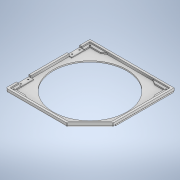
# Autodesk Inventor part: Box_Walls_2
Saved by Autodesk Inventor 2022 (Build 260153000, 153)
## iProperties
Created: 2023-02-27
Part Number: Box_Walls_2
Material: Generic
Document SubType Name: Modeling
Designer: zarek
Density: 1 g/cm^3
Appearance: Default
Author: zarek
Autodesk Inventor part; units mm, degrees
ref_plane "YZ Plane" through (0, 0, 0) normal (1, 0, 0) x (0, 1, 0)
ref_plane "XZ Plane" through (0, 0, 0) normal (0, 1, 0) x (-1, 0, 0)
ref_plane "XY Plane" through (0, 0, 0) normal (0, 0, 1) x (1, 0, 0)
sketch "Sketch1" plane through (0, 0, 0) normal (0, 1, 0) x (-1, 0, 0)
  line L0 (101.6, -101.6) -> (-101.6, -101.6)
  line L1 (-101.6, -101.6) -> (-101.6, 101.6)
  line L2 (-101.6, 101.6) -> (101.6, 101.6)
  line L3 (101.6, 101.6) -> (101.6, -101.6)
  line L4 (96.6, -96.6) -> (-96.6, -96.6)
  line L5 (-96.6, -96.6) -> (-96.6, 96.6)
  line L6 (-96.6, 96.6) -> (96.6, 96.6)
  line L7 (96.6, 96.6) -> (96.6, -96.6)
  line L8 (101.6, 101.6) -> (-40.4, 101.6)
  circle A0 centre (0, 0) radius 88.9
  circle A1 centre (0, 0) radius 109.3376
  line L9 (-40.4, 101.6) -> (-101.6, 40.4)
  line L10 (-45.4, 101.6) -> (-101.6, 45.4)
  line L11 (96.6, 96.6) -> (96.6, 101.6)
  line L12 (-45.4, 101.6) -> (-35.4, 101.6)
  line L13 (-35.4, 101.6) -> (-35.4, 96.6)
  line L14 (-35.4, 96.6) -> (-45.4, 96.6)
  line L15 (-45.4, 96.6) -> (-45.4, 101.6)
  circle A2 centre (0, 0) radius 111.3376
  point P0 (96.6, 51.2168)
  point P1 (101.6, 40.4)
  point P2 (101.6, -40.4)
  point P3 (96.6, -51.2168)
  point P4 (-96.6, 45.4)
  point P5 (-45.4, 96.6)
  dimension "d0" = 203.2
  dimension "d1" = 203.2
  dimension "d2" = 101.6
  dimension "d3" = 101.6
  dimension "d4" = 5
  dimension "d5" = 5
  dimension "d6" = 5
  dimension "d7" = 5
  dimension "d10" = 142
  dimension "d12" = 61.2
  dimension "d14" = 177.8
  dimension "d15" = 5
  dimension "d16" = 5
  dimension "d17" = 10
  dimension "d34" = 2
  constraints: 32 end point, 7 parallel, 6 point on line, 4 perpendicular, 3 centre point, 3 coincident, 3 horizontal, 2 point on circle
  measures "d0" distance between parallel lines of L2 L0
  measures "d1" distance between parallel lines of L1 L3
  measures "d2" distance from line of L0 point (0, 0)
  measures "d3" distance from line of L1 point (0, 0)
  measures "d4" distance between parallel lines of L4 L0
  measures "d5" distance between parallel lines of L1 L5
  measures "d6" distance between parallel lines of L2 L6
  measures "d7" distance between parallel lines of L3 L7
  measures "d10" distance of L2.end L8.end
  measures "d12" distance from line of L1 L8.end
  measures "d14" diameter of A0
  measures "d15" distance of L10.end L9.end
  measures "d16" distance of L10.start L8.end
  measures "d17" distance of L13.end L14.end
  measures "d34" radial gap between concentric circles of A1 A2
extrude "Extrusion1" add sketch "Sketch1" along normal blind 3 contours L0 A2 L4 L7 L3 | L0 A1 L4 A2 | A2 L7 A1 L3 | L0 A1 L4 | A2 L4 A1 L0 | L0 L1 A2 L5 L4 | A2 L7 L4 | L4 A1 L7 A2 | A1 L7 L3 | L4 A1 L5 L9 L6 L7 | A2 L5 A1 L4 | L4 L5 A2 | A1 L7 A2 L3 | A2 L7 L11 L2 L3 | L1 A1 L5 A2 | A1 L6 A2 L7 | A2 L6 L7 | A1 L1 L9 L5 | A1 L2 A2 L6 | L6 L13 L2 A1 | L11 L6 A2 L2 | L9 A1 L10 L5 | L5 L10 L6 L9 | L1 L10 A1 | L6 L9 L2 L13 | L15 A1 L9 | L6 L10 A1 L15 | A1 L15 L2 | A1 L10 L15
sketch "Sketch5" plane through (0, 3, 0) normal (0, 1, 0) x (1, 0, 0)
  line L0 (-101.6, 101.6) -> (101.6, 101.6)
  line L1 (101.6, 101.6) -> (101.6, -101.6)
  line L2 (101.6, -101.6) -> (-101.6, -101.6)
  line L3 (-101.6, -101.6) -> (-101.6, 101.6)
  line L4 (-96.6, 96.6) -> (96.6, 96.6)
  line L5 (96.6, 96.6) -> (96.6, -96.6)
  line L6 (96.6, -96.6) -> (-96.6, -96.6)
  line L7 (-96.6, -96.6) -> (-96.6, 96.6)
  line L8 (-101.6, -101.6) -> (40.4, -101.6)
  circle A0 centre (0, 0) radius 88.9
  circle A1 centre (0, 0) radius 109.3376
  line L9 (40.4, -101.6) -> (101.6, -40.4)
  line L10 (45.4, -101.6) -> (101.6, -45.4)
  line L11 (-96.6, -96.6) -> (-96.6, -101.6)
  line L12 (45.4, -101.6) -> (35.4, -101.6)
  line L13 (35.4, -101.6) -> (35.4, -96.6)
  line L14 (35.4, -96.6) -> (45.4, -96.6)
  line L15 (45.4, -96.6) -> (45.4, -101.6)
  circle A2 centre (0, 0) radius 111.3376
  point P0 (96.6, 101.6)
  point P1 (96.6, 51.2168)
  point P2 (101.6, 40.4)
  point P3 (101.6, -40.4)
  point P4 (96.6, -51.2168)
  point P5 (-96.6, 45.4)
  point P6 (-45.4, 96.6)
  point P7 (-35.4, 101.6)
  point P8 (-55.358, -96.6)
  point P9 (-96.6, -55.358)
  point P10 (-96.6, 55.358)
  point P11 (-55.358, 96.6)
  point P12 (55.358, 96.6)
  point P13 (96.6, 55.358)
  point P14 (96.6, -45.4)
  point P15 (45.4, -96.6)
  dimension "d37" = 203.2
  dimension "d38" = 203.2
  dimension "d39" = 101.6
  dimension "d40" = 101.6
  dimension "d41" = 5
  dimension "d42" = 5
  dimension "d43" = 5
  dimension "d44" = 5
  dimension "d45" = 142
  dimension "d46" = 61.2
  dimension "d47" = 177.8
  dimension "d48" = 5
  dimension "d49" = 5
  dimension "d50" = 10
  dimension "d51" = 2
  constraints: 32 end point, 7 parallel, 6 point on line, 4 perpendicular, 3 centre point, 3 coincident, 2 point on circle
  measures "d37" distance between parallel lines of L2 L0
  measures "d38" distance between parallel lines of L1 L3
  measures "d39" distance from line of L0 point (0, 0)
  measures "d40" distance from line of L1 point (0, 0)
  measures "d41" distance between parallel lines of L4 L0
  measures "d42" distance between parallel lines of L1 L5
  measures "d43" distance between parallel lines of L2 L6
  measures "d44" distance between parallel lines of L3 L7
  measures "d45" distance of L2.end L8.end
  measures "d46" distance from line of L1 L8.end
  measures "d47" diameter of A0
  measures "d48" distance of L10.end L9.end
  measures "d49" distance of L10.start L8.end
  measures "d50" distance of L13.end L14.end
  measures "d51" radial gap between concentric circles of A1 A2
extrude "Extrusion4" add sketch "Sketch5" along normal blind 3 contours L0 A2 L4 L7 L3 | L0 A1 L4 A2 | A2 L7 A1 L3 | L0 A1 L4 | A2 L4 A1 L0 | L0 L1 A2 L5 L4 | A2 L7 L4 | A1 L7 L3 | A2 L7 L11 L2 L3 | L3 A1 L7 A2 | L4 L5 A2 | A2 L6 L7 | L1 A1 L5 A2 | L11 L6 A2 L2 | L6 A1 L2 A2 | A1 L1 L9 L5 | L6 L13 L2 A1 | L9 A1 L10 L5 | L5 L10 L6 L9 | L1 L10 A1 | L6 L9 L2 L13 | L15 A1 L9 | L6 L10 A1 L15 | A1 L15 L2 | L15 A1 L10
sketch "Sketch6" plane through (0, 6, 0) normal (0, 1, 0) x (1, 0, 0)
  line L0 (-101.6, 101.6) -> (101.6, 101.6)
  line L1 (101.6, 101.6) -> (101.6, -101.6)
  line L2 (101.6, -101.6) -> (-101.6, -101.6)
  line L3 (-101.6, -101.6) -> (-101.6, 101.6)
  line L4 (-96.6, 96.6) -> (96.6, 96.6)
  line L5 (96.6, 96.6) -> (96.6, -96.6)
  line L6 (96.6, -96.6) -> (-96.6, -96.6)
  line L7 (-96.6, -96.6) -> (-96.6, 96.6)
  line L8 (-101.6, -101.6) -> (40.4, -101.6)
  circle A0 centre (0, 0) radius 88.9
  circle A1 centre (0, 0) radius 109.3376
  line L9 (40.4, -101.6) -> (101.6, -40.4)
  line L10 (45.4, -101.6) -> (101.6, -45.4)
  line L11 (-96.6, -96.6) -> (-96.6, -101.6)
  line L12 (45.4, -101.6) -> (35.4, -101.6)
  line L13 (35.4, -101.6) -> (35.4, -96.6)
  line L14 (35.4, -96.6) -> (45.4, -96.6)
  line L15 (45.4, -96.6) -> (45.4, -101.6)
  circle A2 centre (0, 0) radius 111.3376
  point P0 (96.6, 101.6)
  point P1 (96.6, 51.2168)
  point P2 (101.6, 40.4)
  point P3 (101.6, -40.4)
  point P4 (96.6, -51.2168)
  point P5 (-96.6, 45.4)
  point P6 (-45.4, 96.6)
  point P7 (-35.4, 101.6)
  point P8 (55.358, 96.6)
  point P9 (96.6, 55.358)
  point P10 (96.6, -45.4)
  point P11 (45.4, -96.6)
  dimension "d54" = 203.2
  dimension "d55" = 203.2
  dimension "d56" = 101.6
  dimension "d57" = 101.6
  dimension "d58" = 5
  dimension "d59" = 5
  dimension "d60" = 5
  dimension "d61" = 5
  dimension "d62" = 142
  dimension "d63" = 61.2
  dimension "d64" = 177.8
  dimension "d65" = 5
  dimension "d66" = 5
  dimension "d67" = 10
  dimension "d68" = 2
  constraints: 32 end point, 7 parallel, 6 point on line, 4 perpendicular, 3 centre point, 3 coincident, 2 point on circle
  measures "d54" distance between parallel lines of L2 L0
  measures "d55" distance between parallel lines of L1 L3
  measures "d56" distance from line of L0 point (0, 0)
  measures "d57" distance from line of L1 point (0, 0)
  measures "d58" distance between parallel lines of L4 L0
  measures "d59" distance between parallel lines of L1 L5
  measures "d60" distance between parallel lines of L2 L6
  measures "d61" distance between parallel lines of L3 L7
  measures "d62" distance of L2.end L8.end
  measures "d63" distance from line of L1 L8.end
  measures "d64" diameter of A0
  measures "d65" distance of L10.end L9.end
  measures "d66" distance of L10.start L8.end
  measures "d67" distance of L13.end L14.end
  measures "d68" radial gap between concentric circles of A1 A2
extrude "Extrusion5" add sketch "Sketch6" along normal blind 3 contours L0 A2 L4 L7 L3 | L0 A1 L4 A2 | A2 L7 A1 L3 | L0 A1 L4 | A2 L4 A1 L0 | L0 L1 A2 L5 L4 | A1 L7 L3 | A2 L7 L11 L2 L3 | L3 A1 L7 A2 | L1 A1 L5 A2 | L11 L6 A2 L2 | L6 A1 L2 A2 | A1 L1 L9 L5 | L6 L13 L2 A1 | L9 A1 L10 L5 | L5 L10 L6 L9 | L1 L10 A1 | L6 L9 L2 L13 | L15 A1 L9 | L6 L10 A1 L15 | A1 L15 L2 | L15 A1 L10
fillet "Fillet6" radius 3.175 5 edges at (-28.1, 0, 101.6) (73.5, 0, 73.5) (101.6, 0, -28.1) (0, 0, -101.6) (-101.6, 0, 0)
sketch "Sketch7" plane through (0, 0, 0) normal (0, -1, 0) x (1, 0, 0)
  line L0 (101.6, 45.4) -> (101.6, -101.6) projected
  line L1 (98.425, 44.0849) -> (98.425, -98.425) projected
  line L2 (101.6, -101.6) -> (98.425, -101.6)
  line L3 (98.425, -101.6) -> (98.425, 39.0849)
  line L4 (98.425, 39.0849) -> (101.6, 39.0849)
  line L5 (101.6, 39.0849) -> (101.6, -101.6)
  line L6 (44.0849, 98.425) -> (98.425, 44.0849) projected
  line L7 (98.425, 44.0849) -> (101.6, 44.0849)
  point P0 (0, 0)
  dimension "d73" = 5
  constraints: 10 end point, 2 horizontal, 2 parallel, 2 point on line, 1 perpendicular
  measures "d73" distance between parallel lines of L4 L7
extrude "Extrusion6" add sketch "Sketch7" against normal blind 3 contours L0 L2 L3 L1 L4
fillet "Fillet7" radius 3.175 1 edges at (100.0125, 0, -101.6)
fillet "Fillet8" radius 3.175 4 edges at (-100.6701, 0.9299, 100.6701) (-101.6, 6.0875, 101.6) (-100.6701, 0.9299, -100.6701) (-101.6, 6.0875, -101.6)
fillet "Fillet9" radius 3.175 4 edges at (100.6701, 0.9299, 45.0148) (101.6, 6.0875, 45.4) (45.0148, 0.9299, 100.6701) (45.4, 6.0875, 101.6)
sketch "Sketch11" plane through (0, 3, 0) normal (0, 1, 0) x (1, 0, 0)
  arc A0 (-101.6, -98.425) -> (-98.425, -101.6) centre (-98.425, -98.425) ccw
  line L0 (44.0849, 101.6) -> (-98.425, 101.6)
  line L1 (-101.6, 98.425) -> (-101.6, -98.425)
  line L2 (-101.6, -46.1) -> (-101.6, -76.6)
  line L3 (-96.6, -96.6) -> (-96.6, 96.6)
  line L4 (-96.6, -46.1) -> (-96.6, -76.6)
  line L5 (-101.6, -76.6) -> (-96.6, -76.6)
  line L6 (-101.6, -46.1) -> (-96.6, -46.1)
  line L7 (-98.425, -101.6) -> (101.6, -101.6)
  line L8 (0, 0) -> (-101.6, 0)
  line L9 (-101.6, 46.1) -> (-101.6, 76.6)
  line L10 (-96.6, 46.1) -> (-96.6, 76.6)
  line L11 (-101.6, 76.6) -> (-96.6, 76.6)
  line L12 (-101.6, 46.1) -> (-96.6, 46.1)
  line L13 (-96.6, -76.6) -> (-90.1, -76.6)
  line L14 (-90.1, -76.6) -> (-90.1, -46.1)
  line L15 (-90.1, -46.1) -> (-96.6, -46.1)
  line L16 (-96.6, -46.1) -> (-96.6, -76.6)
  line L17 (-96.6, 46.1) -> (-90.1, 46.1)
  line L18 (-90.1, 46.1) -> (-90.1, 76.6)
  line L19 (-90.1, 76.6) -> (-96.6, 76.6)
  line L20 (-96.6, 76.6) -> (-96.6, 46.1)
  point P0 (-98.425, 98.425)
  point P1 (46.1, 101.6)
  point P2 (46.1, 96.6)
  point P3 (76.6, 96.6)
  point P4 (76.6, 101.6)
  point P5 (-46.1, 96.6)
  point P6 (-96.6, -46.1)
  point P7 (-101.6, 46.1)
  point P8 (-96.6, 46.1)
  point P9 (-96.6, 76.6)
  point P10 (-101.6, 76.6)
  point P11 (-96.6, 76.6)
  dimension "d97" = 30.5
  dimension "d98" = 25
  dimension "d99" = 5
  dimension "d100" = 6.5
  dimension "d101" = 6.5
  constraints: 42 end point, 5 parallel, 5 symmetric about line, 3 perpendicular, 3 point on line, 2 horizontal, 2 point on circle, 1 centre point, 1 midpoint
  measures "d97" distance between parallel lines of L5 L6
  measures "d98" distance between parallel lines of L5 L7
  measures "d99" distance between parallel lines of L4 L2
  measures "d100" distance of L15.end L14.end
  measures "d101" distance of L19.end L18.end
extrude "Extrusion8" add sketch "Sketch11" along normal up to surface (3 mm away) contours L19 L18 L17 L3 | L15 L14 L13 L3
sketch "Sketch8" plane through (0, 9, 0) normal (0, 1, 0) x (1, 0, 0)
  arc A0 (-101.6, -98.425) -> (-98.425, -101.6) centre (-98.425, -98.425) ccw
  line L0 (44.0849, 101.6) -> (-98.425, 101.6)
  line L1 (-101.6, 98.425) -> (-101.6, -98.425)
  line L2 (-101.6, -46.1) -> (-101.6, -76.6)
  line L3 (-96.6, -96.6) -> (-96.6, 96.6)
  line L4 (-96.6, -46.1) -> (-96.6, -76.6)
  line L5 (-101.6, -76.6) -> (-96.6, -76.6)
  line L6 (-101.6, -46.1) -> (-96.6, -46.1)
  line L7 (-98.425, -101.6) -> (101.6, -101.6)
  line L8 (0, 0) -> (-101.6, 0)
  line L9 (-101.6, 46.1) -> (-101.6, 76.6)
  line L10 (-96.6, 46.1) -> (-96.6, 76.6)
  line L11 (-101.6, 76.6) -> (-96.6, 76.6)
  line L12 (-101.6, 46.1) -> (-96.6, 46.1)
  line L13 (-96.6, -76.6) -> (-90.1, -76.6)
  line L14 (-90.1, -76.6) -> (-90.1, -46.1)
  line L15 (-90.1, -46.1) -> (-96.6, -46.1)
  line L16 (-96.6, -46.1) -> (-96.6, -76.6)
  line L17 (-96.6, 46.1) -> (-90.1, 46.1)
  line L18 (-90.1, 46.1) -> (-90.1, 76.6)
  line L19 (-90.1, 76.6) -> (-96.6, 76.6)
  line L20 (-96.6, 76.6) -> (-96.6, 46.1)
  point P0 (-98.425, 98.425)
  point P1 (46.1, 101.6)
  point P2 (46.1, 96.6)
  point P3 (76.6, 96.6)
  point P4 (76.6, 101.6)
  point P5 (-46.1, 96.6)
  point P6 (-96.6, -46.1)
  point P7 (-101.6, 46.1)
  point P8 (-96.6, 46.1)
  point P9 (-96.6, 76.6)
  point P10 (-101.6, 76.6)
  point P11 (-96.6, 76.6)
  dimension "d77" = 30.5
  dimension "d78" = 25
  dimension "d79" = 5
  dimension "d82" = 6.5
  dimension "d83" = 6.5
  constraints: 42 end point, 5 parallel, 5 symmetric about line, 3 perpendicular, 3 point on line, 2 horizontal, 2 point on circle, 1 centre point, 1 midpoint
  measures "d77" distance between parallel lines of L5 L6
  measures "d78" distance between parallel lines of L5 L7
  measures "d79" distance between parallel lines of L4 L2
  measures "d82" distance of L15.end L14.end
  measures "d83" distance of L19.end L18.end
extrude "Extrusion7" cut sketch "Sketch8" against normal blind 4.2 contours L11 L3 L12 L1 | L19 L18 L17 L3 | L6 L3 L5 L1 | L15 L14 L13 L3
sketch "Sketch10" plane through (0, 4.8, 0) normal (0, 1, 0) x (1, 0, 0)
  line L0 (-90.1, -76.6) -> (-90.1, -46.1)
  line L1 (-101.6, -46.1) -> (-96.6, -46.1)
  line L2 (-90.1, -76.6) -> (-90.1, -46.1)
  line L3 (-90.1, -46.1) -> (-101.6, -46.1)
  line L4 (-101.6, -46.1) -> (-101.6, -76.6)
  line L5 (-101.6, -76.6) -> (-90.1, -76.6)
  line L6 (-96.6, -76.6) -> (-90.1, -76.6)
  line L7 (-91.1, -76.6) -> (-91.1, -46.1)
  line L8 (-91.1, -62.066) -> (-96.35, -62.066)
  line L9 (-96.35, -62.066) -> (-96.35, -71.066)
  line L10 (-96.35, -62.066) -> (-96.35, -53.066)
  circle A0 centre (-96.35, -53.066) radius 1
  circle A1 centre (-96.35, -71.066) radius 1
  line L11 (0, 0) -> (-101.6, 0)
  line L12 (-101.6, 98.425) -> (-101.6, -98.425)
  circle A2 centre (-96.35, 71.066) radius 1
  line L13 (-96.35, 62.066) -> (-96.35, 71.066)
  line L14 (-91.1, 62.066) -> (-96.35, 62.066)
  line L15 (-101.6, 76.6) -> (-90.1, 76.6)
  line L16 (-96.35, 62.066) -> (-96.35, 53.066)
  circle A3 centre (-96.35, 53.066) radius 1
  line L17 (-101.6, 46.1) -> (-96.6, 46.1)
  line L18 (-90.1, 46.1) -> (-101.6, 46.1)
  line L19 (-91.1, 76.6) -> (-91.1, 46.1)
  line L20 (-101.6, 46.1) -> (-101.6, 76.6)
  line L21 (-90.1, 76.6) -> (-90.1, 46.1)
  line L22 (-90.1, 76.6) -> (-90.1, 46.1)
  line L23 (-96.6, 76.6) -> (-90.1, 76.6)
  dimension "d84" = 1
  dimension "d85" = 5.25
  dimension "d86" = 9
  dimension "d87" = 9
  dimension "d88" = 2
  dimension "d89" = 2
  constraints: 48 end point, 15 symmetric about line, 6 point on line, 4 centre point, 4 coincident, 2 parallel, 2 perpendicular, 1 midpoint, 2 other
  measures "d84" distance between parallel lines of L0 L7
  measures "d85" distance of L8.start L8.end
  measures "d86" distance of L8.end L9.end
  measures "d87" distance of L8.end L10.end
  measures "d88" diameter of A0
  measures "d89" diameter of A1
hole "Hinge Holes" at (-96.35, 4.8, -71.066) at (-96.35, 4.8, -53.066) at (-96.35, 4.8, 71.066) at (-96.35, 4.8, 53.066) direction (0, -1, 0) diameter 2.85 depth 4 tip angle 118 countersink diameter 2.9 countersink angle 90 thread size "M3.5x0.6" class "6H" standard "ANSI Metric M Profile"
sketch "Sketch12" plane through (0, 6, 0) normal (0, 1, 0) x (1, 0, 0)
  line L0 (-92, 92) -> (92, 92)
  line L1 (92, 92) -> (92, -92)
  line L2 (92, -92) -> (-92, -92)
  line L3 (-92, -92) -> (-92, 92)
  circle A0 centre (-92, 92) radius 1
  circle A1 centre (92, 92) radius 1
  circle A2 centre (-92, -92) radius 1
  point P0 (0, 0)
  dimension "d104" = 92
  dimension "d105" = 92
  dimension "d106" = 92
  dimension "d107" = 92
  dimension "d108" = 2
  dimension "d109" = 2
  dimension "d110" = 2
  constraints: 8 end point, 3 centre point, 3 coincident, 2 parallel, 1 horizontal, 1 perpendicular
  measures "d104" distance from line of point (0, 0) L0
  measures "d105" distance from line of point (0, 0) L3
  measures "d106" distance from line of point (0, 0) L1
  measures "d107" distance from line of L2 point (0, 0)
  measures "d108" diameter of A0
  measures "d109" diameter of A1
  measures "d110" diameter of A2
hole "Assembly Holes" at (-92, 6, 92) at (-92, 6, -92) at (92, 6, -92) direction (0, -1, 0) diameter 2.85 depth 4 tip angle 118 countersink diameter 2.9 countersink angle 90 thread size "M3.5x0.6" class "6H" standard "ANSI Metric M Profile"
sketch "Sketch15" plane through (0, 3, 0) normal (0, 1, 0) x (1, 0, 0)
  line L0 (-90.17, 90.17) -> (90.17, 90.17)
  line L1 (90.17, 90.17) -> (90.17, -90.17)
  line L2 (90.17, -90.17) -> (-90.17, -90.17)
  line L3 (-90.17, -90.17) -> (-90.17, 90.17)
  line L4 (45.2687, -90.17) -> (90.17, -45.2687)
  point P0 (0, 0)
  dimension "d126" = 90.17
  dimension "d127" = 90.17
  dimension "d128" = 90.17
  dimension "d129" = 90.17
  dimension "d130" = 31.75
  constraints: 10 end point, 2 parallel, 2 point on line, 1 horizontal, 1 perpendicular
  measures "d126" distance from line of L3 point (0, 0)
  measures "d127" distance from line of L1 point (0, 0)
  measures "d128" distance from line of L0 point (0, 0)
  measures "d129" distance from line of L2 point (0, 0)
  measures "d130" distance from line of L4 L1.end
extrude "Extrusion9" cut sketch "Sketch15" along normal blind 10 contours L0 L1 L4 L2 L3
equation "\"d1\" = d0"
equation "\"d2\" = 0.5 * d0"
equation "\"d3\" = 0.5 * d0"
equation "\"d38\" = d37"
equation "\"d39\" = 0.5 * d37"
equation "\"d40\" = 0.5 * d37"
body "Solid1"
